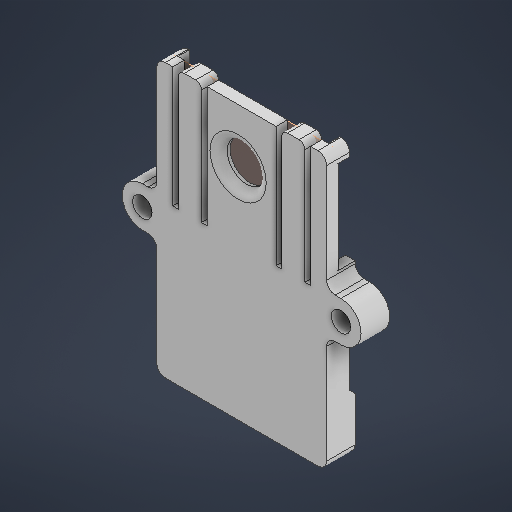
# Autodesk Inventor part: Backplane
Saved by Autodesk Inventor 2025.1 (Build 291241020, 241B)
## iProperties
Created: 2024-09-17
Part Number: Backplane
Material: Generic
Document SubType Name: Modeling
Designer: Sora
Density: 1 g/cm^3
Appearance: Default
Author: Sora
Autodesk Inventor part; units mm, degrees
ref_plane "YZ Plane" through (0, 0, 0) normal (1, 0, 0) x (0, 1, 0)
ref_plane "XZ Plane" through (0, 0, 0) normal (0, 1, 0) x (-1, 0, 0)
ref_plane "XY Plane" through (0, 0, 0) normal (0, 0, 1) x (1, 0, 0)
ref_plane "Work Plane1" through (0, 0, 0) normal (0, 0, 1) x (1, 0, 0)
sketch "Sketch1" plane through (0, 0, 0) normal (0, 0, 1) x (1, 0, 0)
  line L0 (-12.5, -21.5) -> (12.5, -21.5) projected
  line L1 (12.5, -21.5) -> (12.5, 21.5) projected
  line L2 (12.5, 21.5) -> (-12.5, 21.5) projected
  line L3 (-12.5, 21.5) -> (-12.5, -21.5) projected
  circle A0 centre (-9.9, -13.6) radius 0.15 projected
  circle A1 centre (-9.1, -13.6) radius 0.15 projected
  circle A2 centre (-9.7, -12.3) radius 0.15 projected
  circle A3 centre (-8.9, -12.3) radius 0.15 projected
  circle A4 centre (-8.4, -16) radius 0.15 projected
  circle A5 centre (-8.4, -15.2) radius 0.15 projected
  circle A6 centre (-8.4, -14.4) radius 0.15 projected
  circle A7 centre (-8.1, -12.3) radius 0.15 projected
  circle A8 centre (-9.7, -11.5) radius 0.15 projected
  circle A9 centre (-8.9, -11.5) radius 0.15 projected
  circle A10 centre (-8.1, -11.5) radius 0.15 projected
  circle A11 centre (-7, -10.8) radius 0.15 projected
  circle A12 centre (-6.2, -11.3) radius 0.15 projected
  circle A13 centre (-7, -9.8) radius 0.15 projected
  circle A14 centre (-6.5, -8.5) radius 0.15 projected
  circle A15 centre (-6.8, -7.6) radius 0.15 projected
  circle A16 centre (-4.6, -11.3) radius 0.15 projected
  circle A17 centre (-3.8, -10.8) radius 0.15 projected
  circle A18 centre (-3.8, -9.8) radius 0.15 projected
  circle A19 centre (-4.3, -8.5) radius 0.15 projected
  circle A20 centre (-4, -7.6) radius 0.15 projected
  circle A21 centre (-11.4, -5.8) radius 0.15 projected
  circle A22 centre (-11.4, -5) radius 0.15 projected
  circle A23 centre (-10.6, -5.8) radius 0.15 projected
  circle A24 centre (-10.6, -5) radius 0.15 projected
  circle A25 centre (-9.8, -5.8) radius 0.15 projected
  circle A26 centre (-9.8, -5) radius 0.15 projected
  circle A27 centre (-7.2, -6.8) radius 0.15 projected
  circle A28 centre (-6.1, 0.8) radius 0.15 projected
  circle A29 centre (-6.1, 1.8) radius 0.15 projected
  circle A30 centre (-3.6, -6.8) radius 0.15 projected
  circle A31 centre (-4.7, 0.8) radius 0.15 projected
  circle A32 centre (-4.7, 1.8) radius 0.15 projected
  circle A33 centre (-3.9, 1.6) radius 0.15 projected
  circle A34 centre (-2.1, 1.6) radius 0.15 projected
  circle A35 centre (1.6, -10.3) radius 0.15 projected
  circle A36 centre (3.7, -10.8) radius 0.15 projected
  circle A37 centre (3.7, -9.8) radius 0.15 projected
  circle A38 centre (4.6, -11.3) radius 0.15 projected
  circle A39 centre (4.2, -8.5) radius 0.15 projected
  circle A40 centre (3.9, -7.6) radius 0.15 projected
  circle A41 centre (6.2, -11.3) radius 0.15 projected
  circle A42 centre (7.1, -10.8) radius 0.15 projected
  circle A43 centre (7.1, -9.8) radius 0.15 projected
  circle A44 centre (6.6, -8.5) radius 0.15 projected
  circle A45 centre (6.9, -7.6) radius 0.15 projected
  circle A46 centre (2.4, -6.8) radius 0.15 projected
  circle A47 centre (3, -1.6) radius 0.15 projected
  circle A48 centre (3.3, 1.4) radius 0.15 projected
  circle A49 centre (5.6, 1.4) radius 0.15 projected
  circle A50 centre (8.4, -6.8) radius 0.15 projected
  circle A51 centre (9.3, -4.1) radius 0.15 projected
  circle A52 centre (10, -4.1) radius 0.15 projected
  circle A53 centre (10.7, -4.1) radius 0.15 projected
  circle A54 centre (11.4, -4.1) radius 0.15 projected
  circle A55 centre (6.9, 0.6) radius 0.15 projected
  circle A56 centre (10.2, 0.5) radius 0.15 projected
  circle A57 centre (11.1, 1.7) radius 0.15 projected
  circle A58 centre (-11.5, 6.6) radius 0.15 projected
  circle A59 centre (-6.1, 2.8) radius 0.15 projected
  circle A60 centre (-7.4, 4.8) radius 0.15 projected
  circle A61 centre (-11.5, 7.2) radius 0.15 projected
  circle A62 centre (-11.5, 7.8) radius 0.15 projected
  circle A63 centre (-8.9, 9.9) radius 0.15 projected
  circle A64 centre (-8.5, 11) radius 0.15 projected
  circle A65 centre (-7.1, 10.3) radius 0.15 projected
  circle A66 centre (-4.7, 2.8) radius 0.15 projected
  circle A67 centre (-1.9, 2.4) radius 0.15 projected
  circle A68 centre (-1.6, 3.1) radius 0.15 projected
  circle A69 centre (-0.3, 3.1) radius 0.15 projected
  circle A70 centre (-1.1, 8) radius 0.15 projected
  circle A71 centre (-11.2, 11.6) radius 0.15 projected
  circle A72 centre (-10.82, 13.1) radius 0.325 projected
  circle A73 centre (-9.55, 13.1) radius 0.325 projected
  circle A74 centre (-8.6, 12) radius 0.15 projected
  circle A75 centre (-6.3, 13) radius 0.15 projected
  circle A76 centre (-8.1, 15.2) radius 0.15 projected
  circle A77 centre (-9.8, 18.2) radius 0.15 projected
  circle A78 centre (-9.3, 20.2) radius 0.15 projected
  circle A79 centre (-7.4, 16) radius 0.15 projected
  circle A80 centre (-6.6, 20.2) radius 0.15 projected
  circle A81 centre (-5.5, 13) radius 0.15 projected
  circle A82 centre (-3.4, 12.7) radius 0.15 projected
  circle A83 centre (-5.6, 14.3) radius 0.15 projected
  circle A84 centre (-3.5, 15.3) radius 0.15 projected
  circle A85 centre (-0.62, 14.4) radius 0.4 projected
  circle A86 centre (-5.3, 16.3) radius 0.15 projected
  circle A87 centre (-4.2, 17.6) radius 0.15 projected
  circle A88 centre (-2.1, 17) radius 0.15 projected
  circle A89 centre (-1.4, 15.8) radius 0.15 projected
  circle A90 centre (-1, 17.6) radius 0.15 projected
  circle A91 centre (-0.5, 19.3) radius 0.15 projected
  circle A92 centre (1.1, 3.1) radius 0.15 projected
  circle A93 centre (2.2, 2.5) radius 0.15 projected
  circle A94 centre (1, 4.9) radius 0.15 projected
  circle A95 centre (0.9, 5.7) radius 0.15 projected
  circle A96 centre (2.1, 4.6) radius 0.15 projected
  circle A97 centre (3.3, 3.6) radius 0.15 projected
  circle A98 centre (4.4, 2.5) radius 0.15 projected
  circle A99 centre (0.9, 6.7) radius 0.15 projected
  circle A100 centre (1.4, 8.1) radius 0.15 projected
  circle A101 centre (1.4, 9.1) radius 0.15 projected
  circle A102 centre (1.8, 9.7) radius 0.15 projected
  circle A103 centre (3.7, 8.9) radius 0.15 projected
  circle A104 centre (4.6, 8.9) radius 0.15 projected
  circle A105 centre (5.6, 8.9) radius 0.15 projected
  circle A106 centre (0.4, 12.7) radius 0.15 projected
  circle A107 centre (1.7, 13.1) radius 0.15 projected
  circle A108 centre (0.9, 14.4) radius 0.15 projected
  circle A109 centre (2, 15.9) radius 0.15 projected
  line L4 (-14.8, -23.8) -> (14.8, -23.8)
  line L5 (14.8, -23.8) -> (14.8, 23.8)
  line L6 (14.8, 23.8) -> (-14.8, 23.8)
  line L7 (-14.8, 23.8) -> (-14.8, -23.8)
  point P0 (0, 0)
  dimension "d0" = 2.3
  constraints: 8 end point, 3 other
  measures "d0" distance between parallel lines of L3 L7
extrude "Extrusion1" add sketch "Sketch1" along normal blind 2 contours L3 L2 L1 L0 | A0 | A1 | A2 | A3 | A4 | A5 | A6 | A7 | A8 | A9 | A10 | A11 | A12 | A13 | A14 | A15 | A16 | A17 | A18 | A19 | A20 | A21 | A22 | A23 | A24 | A25 | A26 | A27 | A28 | A29 | A30 | A31 | A32 | A33 | A34 | A35 | A36 | A37 | A38 | A39 | A40 | A41 | A42 | A43 | A44 | A45 | A46 | A47 | A48 | A49 | A50 | A51 | A52 | A53 | A54 | A55 | A56 | A57 | A58 | A59 | A60 | A61 | A62 | A63 | A64 | A65 | A66 | A67 | A68 | A69 | A70 | A71 | A72 | A73 | A74 | A75 | A76 | A77 | A78 | A79 | A80 | A81 | A82 | A83 | A84 | A85 | A86 | A87 | A88 | A89 | A90 | A91 | A92 | A93 | A94 | A95 | A96 | A97 | A98 | A99 | A100 | A101 | A102 | A103 | A104 | A105 | A106 | A107 | A108 | A109 | L7 L6 L5 L4
sketch "Sketch2" plane through (0, 0, 0) normal (0, 0, -1) x (-1, 0, 0)
  line L0 (-14.8, -23.8) -> (-14.8, 23.8)
  line L1 (14.8, -23.8) -> (-14.8, -23.8)
  line L2 (14.8, 23.8) -> (14.8, -23.8)
  line L3 (-14.8, 23.8) -> (14.8, 23.8)
  line L4 (-13.1, 22.1) -> (-13.1, -22.1)
  line L5 (-13.1, -22.1) -> (13.1, -22.1)
  line L6 (13.1, -22.1) -> (13.1, 22.1)
  line L7 (13.1, 22.1) -> (-13.1, 22.1)
  line L8 (-7.225, -20.9) -> (-7.225, -14.9)
  line L9 (-7.225, -20.9) -> (-7.85, -20.9)
  line L10 (-7.85, -20.9) -> (-7.85, -17.9)
  line L11 (-7.85, -17.9) -> (-9.35, -17.9)
  line L12 (-9.35, -17.9) -> (-9.35, -13.3)
  line L13 (-9.35, -13.3) -> (-8.55, -13.3)
  line L14 (-8.55, -13.3) -> (-8.55, -14.9)
  line L15 (-8.55, -14.9) -> (-7.225, -14.9)
  line L16 (-3.575, -14.9) -> (-3.575, -20.9)
  line L17 (-3.575, -14.9) -> (-2.25, -14.9)
  line L18 (-2.25, -14.9) -> (-2.25, -13.3)
  line L19 (-2.25, -13.3) -> (-1.45, -13.3)
  line L20 (-1.45, -13.3) -> (-1.45, -17.9)
  line L21 (-1.45, -17.9) -> (-2.95, -17.9)
  line L22 (-2.95, -17.9) -> (-2.95, -20.9)
  line L23 (-2.95, -20.9) -> (-3.575, -20.9)
  line L24 (3.575, -20.9) -> (3.575, -14.9)
  line L25 (3.575, -20.9) -> (2.95, -20.9)
  line L26 (2.95, -20.9) -> (2.95, -17.9)
  line L27 (2.95, -17.9) -> (1.45, -17.9)
  line L28 (1.45, -17.9) -> (1.45, -13.3)
  line L29 (1.45, -13.3) -> (2.25, -13.3)
  line L30 (2.25, -13.3) -> (2.25, -14.9)
  line L31 (2.25, -14.9) -> (3.575, -14.9)
  line L32 (7.225, -14.9) -> (7.225, -20.9)
  line L33 (7.225, -14.9) -> (8.55, -14.9)
  line L34 (8.55, -14.9) -> (8.55, -13.3)
  line L35 (8.55, -13.3) -> (9.35, -13.3)
  line L36 (9.35, -13.3) -> (9.35, -17.9)
  line L37 (9.35, -17.9) -> (7.85, -17.9)
  line L38 (7.85, -17.9) -> (7.85, -20.9)
  line L39 (7.85, -20.9) -> (7.225, -20.9)
  line L40 (-5.7, 9.075) -> (-11.7, 9.075)
  line L41 (-5.7, 9.075) -> (-5.7, 7.75)
  line L42 (-5.7, 7.75) -> (-4.1, 7.75)
  line L43 (-4.1, 7.75) -> (-4.1, 6.95)
  line L44 (-4.1, 6.95) -> (-8.7, 6.95)
  line L45 (-8.7, 6.95) -> (-8.7, 8.45)
  line L46 (-8.7, 8.45) -> (-11.7, 8.45)
  line L47 (-11.7, 8.45) -> (-11.7, 9.075)
  line L48 (-11.7, 18.725) -> (-5.7, 18.725)
  line L49 (-11.7, 18.725) -> (-11.7, 19.35)
  line L50 (-11.7, 19.35) -> (-8.7, 19.35)
  line L51 (-8.7, 19.35) -> (-8.7, 20.85)
  line L52 (-8.7, 20.85) -> (-4.1, 20.85)
  line L53 (-4.1, 20.85) -> (-4.1, 20.05)
  line L54 (-4.1, 20.05) -> (-5.7, 20.05)
  line L55 (-5.7, 20.05) -> (-5.7, 18.725)
  line L56 (-10.85, -22.1) -> (10.85, -22.1)
  line L57 (10.85, -22.1) -> (10.85, -23.8)
  line L58 (10.85, -23.8) -> (-10.85, -23.8)
  line L59 (-10.85, -23.8) -> (-10.85, -22.1)
  line L60 (0, 22.1) -> (0, -22.1) construction
  line L61 (-13.1, 22.1) -> (-13.1, 23.8)
  line L62 (13.1, 22.1) -> (13.1, 23.8)
  line L63 (-13.1, 5.45) -> (-14.8, 5.45)
  line L64 (-13.1, 21.6) -> (-14.8, 21.6)
  line L65 (-11, 23.8) -> (-7, 23.8)
  line L66 (-7, 23.8) -> (-7, 22.1)
  line L67 (-7, 22.1) -> (-11, 22.1)
  line L68 (-11, 22.1) -> (-11, 23.8)
  line L69 (7, 23.8) -> (7, 22.1)
  line L70 (11, 22.1) -> (11, 23.8)
  point P0 (0, 0)
  point P1 (10.85, -22.1)
  point P2 (-11, 22.1)
  point P3 (7, 23.8)
  point P4 (11, 22.1)
  point P5 (11, 23.8)
extrude "Extrusion2" add sketch "Sketch2" along normal blind 2 contours L0 L63 L4 L5 L59 L1 | L0 L3 L61 L4 L64 | L57 L5 L6 L62 L3 L2 L1 | L3 L66 L7 L68 | L70 L7 L69 L3
sketch "Sketch3" plane through (0, 0, 0) normal (0, 0, -1) x (-1, 0, 0)
  circle A0 centre (0.62, 14.4) radius 0.4 projected
  circle A1 centre (0.62, 14.4) radius 3.4
  point P0 (0, 0)
  dimension "d9" = 3
  constraints: 1 centre point
  measures "d9" radial gap between concentric circles of A0 A1
extrude "Extrusion3" cut sketch "Sketch3" against normal through all contours A0 | A1
fillet "Fillet1" radius 1.5 1 edges at (2.78, 14.4, 2)
sketch "Sketch6" plane through (0, 0, 0) normal (0, 0, -1) x (-1, 0, 0)
  line L0 (-11, 22.1) -> (-7, 22.1) projected
  line L1 (-7, 22.1) -> (-7, 23.8) projected
  line L2 (-7, 23.8) -> (-11, 23.8) projected
  line L3 (-11, 23.8) -> (-11, 22.1) projected
  line L4 (7, 22.1) -> (11, 22.1) projected
  line L5 (11, 22.1) -> (11, 23.8) projected
  line L6 (11, 23.8) -> (7, 23.8) projected
  line L7 (7, 23.8) -> (7, 22.1) projected
  line L8 (-11, 23.8) -> (-7, 23.8)
  line L9 (-7, 23.8) -> (-7, 3.8)
  line L10 (-7, 3.8) -> (-11, 3.8)
  line L11 (-11, 3.8) -> (-11, 23.8)
  line L12 (-7, 22.1) -> (-7, 23.8) projected
  line L13 (-7, 23.8) -> (7, 23.8) construction
  line L14 (0, 23.8) -> (0, -23.8) construction
  line L15 (10.85, -23.8) -> (-10.85, -23.8) projected
  line L16 (-12, 24.8) -> (-6, 24.8)
  line L17 (-6, 24.8) -> (-6, 2.8)
  line L18 (-6, 2.8) -> (-12, 2.8)
  line L19 (-12, 2.8) -> (-12, 24.8)
  line L20 (-11, 3.8) -> (-11, 2.8)
  line L21 (-7, 3.8) -> (-7, 2.8)
  line L22 (7, 23.8) -> (7, 3.8)
  line L23 (7, 3.8) -> (11, 3.8)
  line L24 (11, 3.8) -> (11, 23.8)
  line L25 (12, 24.8) -> (6, 24.8)
  line L26 (6, 24.8) -> (6, 2.8)
  line L27 (6, 2.8) -> (12, 2.8)
  line L28 (12, 2.8) -> (12, 24.8)
  line L29 (11, 3.8) -> (11, 2.8)
  line L30 (7, 3.8) -> (7, 2.8)
  point P0 (0, 0)
  dimension "d16" = 20
  dimension "d17" = 1
  constraints: 40 end point, 9 symmetric about line, 4 parallel, 4 perpendicular, 4 point on line, 2 midpoint, 1 collinear, 1 horizontal, 3 other
  measures "d16" distance of L8.end L9.end
  measures "d17" distance between parallel lines of L11 L19
extrude "Extrusion4" cut sketch "Sketch6" against normal through all contours L11 L20 L18 L19 L16 L17 L21 L9 L1 L2 L3 | L22 L30 L27 L26 L25 L28 L29 L24 L5 L6 L7
sketch "Sketch7" plane through (0, 0, -2) normal (0, 0, -1) x (-1, 0, 0)
  line L0 (-14.8, 5.45) -> (-14.8, -23.8) projected
  line L1 (-14.8, -23.8) -> (-10.85, -23.8) projected
  line L2 (-10.85, -23.8) -> (-10.85, -22.1) projected
  line L3 (-10.85, -22.1) -> (-13.1, -22.1) projected
  line L4 (-13.1, -22.1) -> (-13.1, 5.45) projected
  line L5 (-13.1, 5.45) -> (-14.8, 5.45) projected
  line L6 (14.8, 23.8) -> (13.1, 23.8) projected
  line L7 (13.1, 23.8) -> (13.1, -22.1) projected
  line L8 (13.1, -22.1) -> (10.85, -22.1) projected
  line L9 (10.85, -22.1) -> (10.85, -23.8) projected
  line L10 (10.85, -23.8) -> (14.8, -23.8) projected
  line L11 (14.8, -23.8) -> (14.8, 23.8) projected
  line L12 (10.85, -23.8) -> (-10.85, -23.8) projected
  line L13 (0, -23.8) -> (0, 23.8) construction
  line L14 (-6, 23.8) -> (6, 23.8) projected
  line L15 (-14.8, -23.8) -> (-10.85, -23.8) projected
  line L16 (-14.8, -23.8) -> (-10.85, -23.8)
  line L17 (-10.85, -23.8) -> (-10.85, -14.6)
  line L18 (-10.85, -14.6) -> (-14.8, -14.6)
  line L19 (-14.8, -14.6) -> (-14.8, -23.8)
  line L20 (-10.85, -23.8) -> (-10.85, -22.1) projected
  line L21 (10.85, -23.8) -> (10.85, -14.6)
  line L22 (10.85, -14.6) -> (14.8, -14.6)
  line L23 (-11, 22.1) -> (-7, 22.1) projected
  line L24 (-7, 22.1) -> (-7, 23.8) projected
  line L25 (-7, 23.8) -> (-11, 23.8) projected
  line L26 (-11, 23.8) -> (-11, 22.1) projected
  line L27 (7, 22.1) -> (11, 22.1) projected
  line L28 (11, 22.1) -> (11, 23.8) projected
  line L29 (11, 23.8) -> (7, 23.8) projected
  line L30 (7, 23.8) -> (7, 22.1) projected
  line L31 (-7, 2.8) -> (-7, 22.1) projected
  line L32 (-11, 22.1) -> (-7, 22.1)
  line L33 (-7, 22.1) -> (-7, 21.1)
  line L34 (-7, 21.1) -> (-11, 21.1)
  line L35 (-11, 21.1) -> (-11, 22.1)
  line L36 (7, 22.1) -> (7, 21.1)
  line L37 (7, 21.1) -> (11, 21.1)
  line L38 (11, 21.1) -> (11, 22.1)
  line L39 (-13.1, 5.45) -> (-12.1, 5.45)
  line L40 (-12.1, 5.45) -> (-12.1, -4.55)
  line L41 (-12.1, -4.55) -> (-13.1, -4.55)
  line L42 (-13.1, -4.55) -> (-13.1, 5.45)
  line L43 (13.1, 5.45) -> (12.1, 5.45)
  line L44 (12.1, 5.45) -> (12.1, -4.55)
  line L45 (12.1, -4.55) -> (13.1, -4.55)
  line L46 (-13.1, -4.55) -> (-14.8, -4.55)
  line L47 (13.1, 5.45) -> (14.8, 5.45)
  line L48 (13.1, -4.55) -> (14.8, -4.55)
  point P0 (0, 0)
  point P1 (-11.975, -22.1)
  point P2 (14.8, -14.6)
  point P3 (-14.8, -14.6)
  dimension "d20" = 7.5
  dimension "d21" = 1
  dimension "d44" = 1
  dimension "d45" = 10
  constraints: 48 end point, 10 symmetric about line, 6 parallel, 5 perpendicular, 5 point on line, 3 horizontal, 3 midpoint, 1 collinear
  measures "d20" distance from line of point (-11.975, -22.1) L18
  measures "d21" distance between parallel lines of L32 L34
  measures "d44" distance of L40.end L41.end
  measures "d45" distance of L39.end L40.end
extrude "Extrusion5" add sketch "Sketch7" along normal blind 1 contours L5 L4 L46 L0 | L39 L40 L41 L4 | L18 L4 L3 L2 L1 L0 | L18 L17 L3 L4 | L11 L48 L7 L47 | L7 L45 L44 L43 | L11 L10 L9 L8 L7 L22 | L7 L8 L21 L22
chamfer "Chamfer1" distance 1 angle 45 5 edges at (13.95, -14.6, -2) (-13.95, -14.6, -2) (13.95, -4.55, -2) (-13.95, -4.55, -2) (-13.95, 5.45, -2)
fillet "Fillet2" radius 1 4 edges at (11, 23.8, 0) (7, 23.8, 0) (-7, 23.8, 0) (-11, 23.8, 0)
fillet "Fillet3" radius 1.5 4 edges at (-14.8, -23.8, -0.5) (14.8, -23.8, -0.5) (14.8, 23.8, 0) (-14.8, 23.8, 0)
chamfer "Chamfer2" distance 1 angle 45 6 edges at (10.85, -14.6, -2.5) (-10.85, -14.6, -2.5) (12.1, -4.55, -2.5) (12.1, 5.45, -2.5) (-12.1, 5.45, -2.5) (-12.1, -4.55, -2.5)
sketch "Sketch9" plane through (0, 0, 2) normal (0, 0, 1) x (1, 0, 0)
  circle A0 centre (-0.62, 14.4) radius 4.9 projected
  arc A1 (-13.3, 23.8) -> (-14.8, 22.3) centre (-13.3, 22.3) ccw projected
  line L0 (-14.8, 22.3) -> (-14.8, -22.3) projected
  arc A2 (-14.8, -22.3) -> (-13.3, -23.8) centre (-13.3, -22.3) ccw projected
  line L1 (-13.3, -23.8) -> (13.3, -23.8) projected
  arc A3 (13.3, -23.8) -> (14.8, -22.3) centre (13.3, -22.3) ccw projected
  line L2 (14.8, -22.3) -> (14.8, 22.3) projected
  arc A4 (14.8, 22.3) -> (13.3, 23.8) centre (13.3, 22.3) ccw projected
  line L3 (13.3, 23.8) -> (12, 23.8) projected
  line L4 (12, 23.8) -> (12, 2.8) projected
  line L5 (12, 2.8) -> (11, 2.8) projected
  line L6 (11, 2.8) -> (11, 22.8) projected
  arc A5 (11, 22.8) -> (10, 23.8) centre (10, 22.8) ccw projected
  line L7 (10, 23.8) -> (8, 23.8) projected
  arc A6 (8, 23.8) -> (7, 22.8) centre (8, 22.8) ccw projected
  line L8 (7, 22.8) -> (7, 2.8) projected
  line L9 (7, 2.8) -> (6, 2.8) projected
  line L10 (6, 2.8) -> (6, 23.8) projected
  line L11 (6, 23.8) -> (-6, 23.8) projected
  line L12 (-6, 23.8) -> (-6, 2.8) projected
  line L13 (-6, 2.8) -> (-7, 2.8) projected
  line L14 (-7, 2.8) -> (-7, 22.8) projected
  arc A7 (-7, 22.8) -> (-8, 23.8) centre (-8, 22.8) ccw projected
  line L15 (-8, 23.8) -> (-10, 23.8) projected
  arc A8 (-10, 23.8) -> (-11, 22.8) centre (-10, 22.8) ccw projected
  line L16 (-11, 22.8) -> (-11, 2.8) projected
  line L17 (-11, 2.8) -> (-12, 2.8) projected
  line L18 (-12, 2.8) -> (-12, 23.8) projected
  line L19 (-12, 23.8) -> (-13.3, 23.8) projected
  line L20 (-17.3, 0) -> (17.3, 0) construction
  line L21 (-17.3, -3.5) -> (17.3, -3.5)
  line L22 (17.3, 3.5) -> (-17.3, 3.5)
  arc A9 (-17.3, 3.5) -> (-17.3, -3.5) centre (-17.3, 0) ccw
  arc A10 (17.3, -3.5) -> (17.3, 3.5) centre (17.3, 0) ccw
  point P0 (0, 0)
  point P1 (14.8, 3.5)
  point P2 (14.8, -3.5)
  point P3 (-14.8, -3.5)
  point P4 (-14.8, 3.5)
  dimension "d32" = 7
  dimension "d33" = 2.5
  constraints: 8 end point, 4 point on circle, 4 tangent, 2 centre point, 1 horizontal, 1 midpoint, 1 parallel
  measures "d32" diameter of A10
  measures "d33" distance from line of L2 L20.end
extrude "Extrusion6" add sketch "Sketch9" against normal up to surface (5 mm away) contours L0 L21 A9 L22 | L2 L22 A10 L21
fillet "Fillet4" radius 1.5 4 edges at (14.8, 3.5, -0.5) (14.8, -3.5, -0.5) (-14.8, -3.5, -0.5) (-14.8, 3.5, -0.5)
sketch "Sketch10" plane through (0, 0, 2) normal (0, 0, 1) x (1, 0, 0)
  circle A0 centre (-0.62, 14.4) radius 4.9 projected
  arc A1 (-13.3, 23.8) -> (-14.8, 22.3) centre (-13.3, 22.3) ccw projected
  line L0 (-14.8, 22.3) -> (-14.8, 5) projected
  arc A2 (-16.3, 3.5) -> (-14.8, 5) centre (-16.3, 5) ccw projected
  line L1 (-16.3, 3.5) -> (-17.3, 3.5) projected
  arc A3 (-17.3, 3.5) -> (-17.3, -3.5) centre (-17.3, 0) ccw projected
  line L2 (-17.3, -3.5) -> (-16.3, -3.5) projected
  arc A4 (-14.8, -5) -> (-16.3, -3.5) centre (-16.3, -5) ccw projected
  line L3 (-14.8, -5) -> (-14.8, -22.3) projected
  arc A5 (-14.8, -22.3) -> (-13.3, -23.8) centre (-13.3, -22.3) ccw projected
  line L4 (-13.3, -23.8) -> (13.3, -23.8) projected
  arc A6 (13.3, -23.8) -> (14.8, -22.3) centre (13.3, -22.3) ccw projected
  line L5 (14.8, -22.3) -> (14.8, -5) projected
  arc A7 (16.3, -3.5) -> (14.8, -5) centre (16.3, -5) ccw projected
  line L6 (16.3, -3.5) -> (17.3, -3.5) projected
  arc A8 (17.3, -3.5) -> (17.3, 3.5) centre (17.3, 0) ccw projected
  line L7 (17.3, 3.5) -> (16.3, 3.5) projected
  arc A9 (14.8, 5) -> (16.3, 3.5) centre (16.3, 5) ccw projected
  line L8 (14.8, 5) -> (14.8, 22.3) projected
  arc A10 (14.8, 22.3) -> (13.3, 23.8) centre (13.3, 22.3) ccw projected
  line L9 (13.3, 23.8) -> (12, 23.8) projected
  line L10 (12, 23.8) -> (12, 2.8) projected
  line L11 (12, 2.8) -> (11, 2.8) projected
  line L12 (11, 2.8) -> (11, 22.8) projected
  arc A11 (11, 22.8) -> (10, 23.8) centre (10, 22.8) ccw projected
  line L13 (10, 23.8) -> (8, 23.8) projected
  arc A12 (8, 23.8) -> (7, 22.8) centre (8, 22.8) ccw projected
  line L14 (7, 22.8) -> (7, 2.8) projected
  line L15 (7, 2.8) -> (6, 2.8) projected
  line L16 (6, 2.8) -> (6, 23.8) projected
  line L17 (6, 23.8) -> (-6, 23.8) projected
  line L18 (-6, 23.8) -> (-6, 2.8) projected
  line L19 (-6, 2.8) -> (-7, 2.8) projected
  line L20 (-7, 2.8) -> (-7, 22.8) projected
  arc A13 (-7, 22.8) -> (-8, 23.8) centre (-8, 22.8) ccw projected
  line L21 (-8, 23.8) -> (-10, 23.8) projected
  arc A14 (-10, 23.8) -> (-11, 22.8) centre (-10, 22.8) ccw projected
  line L22 (-11, 22.8) -> (-11, 2.8) projected
  line L23 (-11, 2.8) -> (-12, 2.8) projected
  line L24 (-12, 2.8) -> (-12, 23.8) projected
  line L25 (-12, 23.8) -> (-13.3, 23.8) projected
  point P0 (0, 0)
hole "Hole1" at (-17.3, 0, 2) at (17.3, 0, 2) direction (0, 0, -1) diameter 3.4 end through all clearance for "Socket Head Cap Screw" size "M3" standard "Ansi Metric M Profile"
sketch "Sketch11" plane through (0, 0, -2) normal (0, 0, -1) x (-1, 0, 0)
  arc A0 (-7, 22.8) -> (-8, 23.8) centre (-8, 22.8) ccw projected
  line L0 (-8, 23.8) -> (-10, 23.8) projected
  arc A1 (-10, 23.8) -> (-11, 22.8) centre (-10, 22.8) ccw projected
  line L1 (-11, 22.8) -> (-11, 22.1) projected
  line L2 (-11, 22.1) -> (-7, 22.1) projected
  line L3 (-7, 22.1) -> (-7, 22.8) projected
  arc A2 (11, 22.8) -> (10, 23.8) centre (10, 22.8) ccw projected
  line L4 (10, 23.8) -> (8, 23.8) projected
  arc A3 (8, 23.8) -> (7, 22.8) centre (8, 22.8) ccw projected
  line L5 (7, 22.8) -> (7, 22.1) projected
  line L6 (7, 22.1) -> (11, 22.1) projected
  line L7 (11, 22.1) -> (11, 22.8) projected
  point P0 (0, 0)
extrude "Extrusion7" cut sketch "Sketch11" against normal blind 1
body "Solid1"
